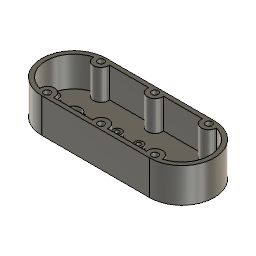
robosoc_motor_case_with_hole (Autodesk Fusion 360 design; units mm, degrees)
part number: 2025-12-10-15-49-31-313
Autodesk Fusion 360 part; units mm, degrees
sketch "Sketch1" plane through (0, 0, 0) normal (0, 0, 1) x (1, 0, 0)
  line L0 (15, 0) -> (65, 0)
  line L1 (65, 30) -> (15, 30)
  arc A0 (15, 30) -> (0, 15) centre (15, 15) ccw
  arc A1 (0, 15) -> (15, 0) centre (15, 15) ccw
  arc A2 (80, 15) -> (65, 30) centre (65, 15) ccw
  arc A3 (65, 0) -> (80, 15) centre (65, 15) ccw
  line L2 (15, 15) -> (65, 15) construction
  line L3 (15, 15) -> (15, 27.5) construction
  line L4 (65, 15) -> (65, 27.5) construction
  line L5 (15, 27.5) -> (40, 27.5) construction
  circle A4 centre (15, 27.5) radius 1.5
  circle A5 centre (40, 27.5) radius 1.5
  circle A6 centre (65, 27.5) radius 1.5
  circle A7 centre (15, 2.5) radius 1.5
  circle A8 centre (40, 2.5) radius 1.5
  circle A9 centre (65, 2.5) radius 1.5
  point P0 (80, 0)
  point P1 (0, 30)
  dimension "d1" = 80
  dimension "d2" = 30
  dimension "d3" = 15
  dimension "d4" = 15
  dimension "d5" = 15
  dimension "d6" = 15
  dimension "d7" = 12.5
  dimension "d8" = 12.5
  dimension "d9" = 25
  dimension "d11" = 3
  dimension "d12" = 3
  dimension "d13" = 3
  constraint horizontal L0
  constraint horizontal L1
  constraint coincident P1 L1
  constraint tangent L1 A0
  constraint coincident origin L0
  constraint tangent L0 A1
  constraint coincident A0.end A1.start
  constraint tangent L1 A2
  constraint coincident P0 L0
  constraint tangent L0 A3
  constraint coincident A2.start A3.end
  constraint coincident A0.centre A1.centre
  constraint coincident A2.centre A3.centre
  constraint perpendicular L1 L3
  constraint perpendicular L2 L4
  constraint perpendicular L3 L5
  constraint coincident L3.end L5.start
  constraint coincident L5.end A5.centre
  constraint coincident L4.end A6.centre
  constraint symmetric L2 A4 A7
  constraint symmetric L2 A5 A8
  constraint symmetric L2 A6 A9
  measures "d1" distance of origin P0
  measures "d2" distance of origin P1
  measures "d3" radius of A0
  measures "d4" radius of A1
  measures "d5" radius of A2
  measures "d6" radius of A3
  measures "d7" distance of A0.centre L3.end
  measures "d8" distance of A2.centre L4.end
  measures "d9" distance of L3.end L5.end
  measures "d11" diameter of A4
  measures "d12" diameter of A5
  measures "d13" diameter of A6
extrude "Extrude1" add sketch "Sketch1" along normal blind 16
shell "Shell1" thickness 2 removed faces 1 at (23.6999, 18.8266, 16)
sketch "Sketch2" plane through (0, 0, 2) normal (0, 0, 1) x (-1, 0, 0)
  arc A0 (-68.4999, -2.48) -> (-61.5359, -2) centre (-65, -2.5) ccw
  arc A1 (-68.4999, -2.48) -> (-68.4999, -27.52) centre (-65, -15) ccw
  arc A2 (-61.5359, -28) -> (-68.4999, -27.52) centre (-65, -27.5) ccw
  line L0 (-61.5359, -28) -> (-43.4641, -28)
  arc A3 (-36.5359, -28) -> (-43.4641, -28) centre (-40, -27.5) ccw
  line L1 (-36.5359, -28) -> (-18.4641, -28)
  arc A4 (-11.5001, -27.52) -> (-18.4641, -28) centre (-15, -27.5) ccw
  arc A5 (-11.5001, -27.52) -> (-11.5001, -2.48) centre (-15, -15) ccw
  arc A6 (-18.4641, -2) -> (-11.5001, -2.48) centre (-15, -2.5) ccw
  line L2 (-18.4641, -2) -> (-36.5359, -2)
  arc A7 (-43.4641, -2) -> (-36.5359, -2) centre (-40, -2.5) ccw
  line L3 (-43.4641, -2) -> (-61.5359, -2)
  line L4 (-15, -2.5) -> (-15, -27.5) construction
  arc A8 (-17.9038, -13.5405) -> (-17.9038, -16.4595) centre (-18.25, -15) ccw
  arc A9 (-17.9038, -16.4595) -> (-17.9038, -13.5405) centre (-15, -15) ccw
  arc A10 (-62.0962, -13.5405) -> (-62.0962, -16.4595) centre (-65, -15) ccw
  arc A11 (-62.0962, -16.4595) -> (-62.0962, -13.5405) centre (-61.75, -15) ccw
  line L5 (-15, -15) -> (-35, -15) construction
  line L6 (-15, -15) -> (-6, -15) construction
  line L7 (-65, -15) -> (-45, -15) construction
  line L8 (-65, -15) -> (-74, -15) construction
  circle A12 centre (-6, -15) radius 1
  circle A13 centre (-35, -15) radius 1
  circle A14 centre (-74, -15) radius 1
  circle A15 centre (-45, -15) radius 1
  circle A16 centre (-35, -15) radius 2
  circle A17 centre (-6, -15) radius 2
  circle A18 centre (-45, -15) radius 2
  circle A19 centre (-74, -15) radius 2
  dimension "d17" = 6.5
  dimension "d18" = 6.5
  dimension "d19" = 3
  dimension "d20" = 3
  dimension "d22" = 20
  dimension "d23" = 9
  dimension "d24" = 20
  dimension "d25" = 9
  dimension "d26" = 2
  dimension "d27" = 2
  dimension "d29" = 2
  dimension "d31" = 2
  dimension "d32" = 1
  dimension "d33" = 1
  dimension "d34" = 1
  dimension "d35" = 1
  constraint coincident A6.centre L4.start
  constraint coincident A4.centre L4.end
  constraint concentric A5 A9
  constraint coincident A5.centre A9.centre
  constraint perpendicular L4 L5
  constraint perpendicular L4 L6
  constraint coincident A1.centre A10.centre
  constraint parallel L1 L7
  constraint parallel L7 L8
  constraint coincident L6.end A12.centre
  constraint coincident L5.end A13.centre
  constraint coincident L8.end A14.centre
  constraint coincident L7.end A15.centre
  measures "d17" diameter of A9
  measures "d18" diameter of A10
  measures "d19" diameter of A8
  measures "d20" diameter of A11
  measures "d22" distance of A5.centre L5.end
  measures "d23" distance of A5.centre L6.end
  measures "d24" distance of A1.centre L7.end
  measures "d25" distance of A1.centre L8.end
  measures "d26" diameter of A12
  measures "d27" diameter of A13
  measures "d29" diameter of A14
  measures "d31" diameter of A15
  measures "d32" distance of A13
  measures "d33" distance of A12
  measures "d34" distance of A15
  measures "d35" distance of A14
extrude "Extrude2" cut sketch "Sketch2" against normal through all contours A8 A9 | A10 A11
extrude "Extrude3" add sketch "Sketch2" along normal blind 2 contours A16 | A17 | A18 | A19
